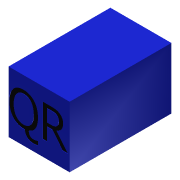
# Autodesk Inventor part: Container 2 2 2 and half color 5
Saved by Autodesk Inventor 2015 (Build 190159000, 159)
## iProperties
Created: 2015-03-07
Part Number: Container 2 2 2 and half color 5
Material: Generic
Document SubType Name: Modeling
Designer: Vukica
Density: 1 g/cm^3
Appearance: Blue - Wall Paint - Glossy
Author: Vukica
Autodesk Inventor part; units mm, degrees
ref_plane "YZ Plane" through (0, 0, 0) normal (1, 0, 0) x (0, 1, 0)
ref_plane "XZ Plane" through (0, 0, 0) normal (0, 1, 0) x (-1, 0, 0)
ref_plane "XY Plane" through (0, 0, 0) normal (0, 0, 1) x (1, 0, 0)
sketch "Sketch1" plane through (0, 0, 0) normal (0, 0, 1) x (1, 0, 0)
  line L0 (0, 0) -> (38.1, 0)
  line L1 (38.1, 0) -> (38.1, 38.1)
  line L2 (38.1, 38.1) -> (0, 38.1)
  line L3 (0, 38.1) -> (0, 0)
  dimension "d0" = 38.1
  dimension "d1" = 38.1
  constraints: 8 end point, 2 parallel, 1 horizontal, 1 perpendicular
  measures "d0" distance of L1.end L2.end
  measures "d1" distance of L2.end L0.start
extrude "Extrusion1" add sketch "Sketch1" along normal blind 63.5
sketch "Sketch2" plane through (0, 0, 63.5) normal (0, 0, 1) x (1, 0, 0)
  line L0 (-0.5245, 30.1882) -> (22.6731, 30.1882) construction
  line L1 (22.6731, 30.1882) -> (22.6731, 13.8758) construction
  line L2 (22.6731, 13.8758) -> (-0.5245, 13.8758) construction
  line L3 (-0.5245, 13.8758) -> (-0.5245, 30.1882) construction
  spline S0 degree 2 poles (18.4123, 4.4671) (17.6713, 4.286) (16.0575, 4.0884) (15.2507, 4.0884) knots 0 0 0 1 2 2 2
  spline S1 degree 2 poles (15.2507, 4.0884) (12.9618, 4.0884) (10.113, 6.6407) (9.9813, 9.0119) knots 0 0 0 1 2 2 2
  spline S2 degree 2 poles (9.9813, 9.0119) (9.8002, 9.0119) (9.4873, 9.0119) (9.3556, 9.0119) knots 0 0 0 1 2 2 2
  spline S3 degree 2 poles (9.3556, 9.0119) (7.2972, 9.0119) (3.9874, 10.4116) (2.8018, 11.7784) knots 0 0 0 1 2 2 2
  spline S4 degree 2 poles (2.8018, 11.7784) (1.6326, 13.1286) (0.3812, 17.0807) (0.3812, 19.5836) knots 0 0 0 1 2 2 2
  spline S5 degree 2 poles (0.3812, 19.5836) (0.3812, 22.1524) (1.6491, 26.0386) (2.8183, 27.4218) knots 0 0 0 1 2 2 2
  spline S6 degree 2 poles (2.8183, 27.4218) (4.0039, 28.7885) (7.3137, 30.1882) (9.3556, 30.1882) knots 0 0 0 1 2 2 2
  spline S7 degree 2 poles (9.3556, 30.1882) (11.4304, 30.1882) (14.7567, 28.7391) (15.9093, 27.4218) knots 0 0 0 1 2 2 2
  spline S8 degree 2 poles (15.9093, 27.4218) (17.062, 26.088) (18.3464, 22.1195) (18.3464, 19.5836) knots 0 0 0 1 2 2 2
  spline S9 degree 2 poles (18.3464, 19.5836) (18.3464, 15.6316) (15.2671, 10.4939) (12.583, 9.5883) knots 0 0 0 1 2 2 2
  spline S10 degree 2 poles (12.583, 9.5883) (12.6489, 8.8308) (13.0441, 7.6123) (13.357, 7.2665) knots 0 0 0 1 2 2 2
  spline S11 degree 2 poles (13.357, 7.2665) (13.7357, 6.8383) (14.7731, 6.4431) (15.6953, 6.4431) knots 0 0 0 1 2 2 2
  spline S12 degree 2 poles (15.6953, 6.4431) (16.2387, 6.4431) (17.7207, 6.7889) (18.05, 6.9207) knots 0 0 0 1 2 2 2
  line L4 (18.05, 6.9207) -> (18.4123, 6.9207)
  line L5 (18.4123, 6.9207) -> (18.4123, 4.4671)
  spline S13 degree 2 poles (15.5306, 19.5836) (15.5306, 21.609) (14.6579, 24.7212) (13.8675, 25.7422) knots 0 0 0 1 2 2 2
  spline S14 degree 2 poles (13.8675, 25.7422) (13.0606, 26.7961) (10.7882, 27.8499) (9.372, 27.8499) knots 0 0 0 1 2 2 2
  spline S15 degree 2 poles (9.372, 27.8499) (7.9065, 27.8499) (5.6999, 26.829) (4.8601, 25.7422) knots 0 0 0 1 2 2 2
  spline S16 degree 2 poles (4.8601, 25.7422) (4.0533, 24.7048) (3.197, 21.5596) (3.197, 19.5836) knots 0 0 0 1 2 2 2
  spline S17 degree 2 poles (3.197, 19.5836) (3.197, 15.5822) (6.5562, 11.3173) (9.372, 11.3173) knots 0 0 0 1 2 2 2
  spline S18 degree 2 poles (9.372, 11.3173) (12.1878, 11.3173) (15.5306, 15.5822) (15.5306, 19.5836) knots 0 0 0 1 2 2 2
  line L6 (37.0362, 9.4401) -> (33.5288, 9.4401)
  line L7 (33.5288, 9.4401) -> (27.1067, 17.5253)
  line L8 (27.1067, 17.5253) -> (24.011, 17.5253)
  line L9 (24.011, 17.5253) -> (24.011, 9.4401)
  line L10 (24.011, 9.4401) -> (21.3104, 9.4401)
  line L11 (21.3104, 9.4401) -> (21.3104, 29.7601)
  line L12 (21.3104, 29.7601) -> (26.5469, 29.7601)
  spline S19 degree 2 poles (26.5469, 29.7601) (28.2924, 29.7601) (30.6471, 29.3813) (31.7174, 28.6897) knots 0 0 0 1 2 2 2
  spline S20 degree 2 poles (31.7174, 28.6897) (32.7878, 27.9981) (34.0228, 25.841) (34.0228, 24.2437) knots 0 0 0 1 2 2 2
  spline S21 degree 2 poles (34.0228, 24.2437) (34.0228, 22.0207) (31.7504, 19.0073) (29.8073, 18.2827) knots 0 0 0 1 2 2 2
  line L13 (29.8073, 18.2827) -> (37.0362, 9.4401)
  spline S22 degree 2 poles (31.207, 24.0296) (31.207, 24.9188) (30.5812, 26.2856) (29.9226, 26.7302) knots 0 0 0 1 2 2 2
  spline S23 degree 2 poles (29.9226, 26.7302) (29.3462, 27.1089) (27.8148, 27.4218) (26.6951, 27.4218) knots 0 0 0 1 2 2 2
  line L14 (26.6951, 27.4218) -> (24.011, 27.4218)
  line L15 (24.011, 27.4218) -> (24.011, 19.7812)
  line L16 (24.011, 19.7812) -> (26.3822, 19.7812)
  spline S24 degree 2 poles (26.3822, 19.7812) (27.5513, 19.7812) (29.4121, 20.1929) (30.0543, 20.8351) knots 0 0 0 1 2 2 2
  spline S25 degree 2 poles (30.0543, 20.8351) (30.6471, 21.395) (31.207, 22.9758) (31.207, 24.0296) knots 0 0 0 1 2 2 2
  point P0 (0, 0)
  constraints: 2 other
extrude "Extrusion2" cut sketch "Sketch2" against normal blind 0.254
equation "\"d1\" = d0"
body "Solid1"
